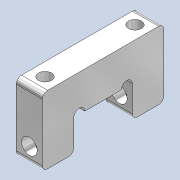
# Autodesk Inventor part: ウィング土台
Saved by Autodesk Inventor 2020 (Build 240168000, 168)
## iProperties
Created: 2020-10-30
Part Number: ウィング土台
Material: アルミニウム 2014-T4
Document SubType Name: Modeling
Designer: AA19065
Density: 2.8 g/cm^3
Appearance: サテン
Author: AA19065
Autodesk Inventor part; units mm, degrees
ref_plane "YZ Plane" through (0, 0, 0) normal (1, 0, 0) x (0, 1, 0)
ref_plane "XZ Plane" through (0, 0, 0) normal (0, 1, 0) x (-1, 0, 0)
ref_plane "XY Plane" through (0, 0, 0) normal (0, 0, 1) x (1, 0, 0)
sketch "スケッチ1" plane through (0, 0, 0) normal (1, 0, 0) x (0, 1, 0)
  line L0 (7, 5.6) -> (0, 5.6)
  line L1 (0, 5.6) -> (0, -5.6)
  line L2 (0, -5.6) -> (7, -5.6)
  line L3 (7, -5.6) -> (7, 5.6)
  line L4 (7, 5.6) -> (-6, 5.6)
  line L5 (-6, 5.6) -> (-6, 13.6)
  line L6 (-6, 13.6) -> (7, 13.6)
  line L7 (7, 13.6) -> (7, 5.6)
  line L8 (7, -5.6) -> (-6, -5.6)
  line L9 (-6, -5.6) -> (-6, -13.6)
  line L10 (-6, -13.6) -> (7, -13.6)
  line L11 (7, -13.6) -> (7, -5.6)
  arc A0 (0, 3.5) -> (0, 5.6) centre (0, 4.55) ccw
  arc A1 (0, -5.6) -> (0, -3.5) centre (0, -4.55) ccw
  point P0 (0, 0)
  point P1 (0, 0)
  point P2 (0, 5.6)
  point P3 (0, 5.6)
  dimension "d0" = 7
  dimension "d1" = 11.2
  dimension "d2" = 13
  dimension "d3" = 13
  dimension "d4" = 8
  dimension "d5" = 8
  dimension "d8" = 1.05
  constraints: 24 end point, 6 parallel, 4 point on circle, 3 horizontal, 3 perpendicular, 2 centre point, 2 point on line, 2 tangent, 1 coincident, 1 equal radius, 1 midpoint
  measures "d0" distance of L2.end L1.end
  measures "d1" distance of L1.end L0.end
  measures "d2" distance of L5.end L6.end
  measures "d3" distance of L10.end L9.end
  measures "d4" distance of L4.end L5.end
  measures "d5" distance of L8.end L9.end
  measures "d8" radius of A0
extrude "押し出し1" add sketch "スケッチ1" along normal blind 5 contours L3 L2 A1 L1 A0 L0 | L0 L4 L5 L6 L7 | L11 L10 L9 L8 L2
sketch "スケッチ2" plane through (0, 7, 13.6) normal (0, 1, 0) x (1, 0, 0)
  line L0 (0, 27.2) -> (0, 0) projected
  line L1 (0, 0) -> (5, 0) projected
  line L2 (5, 27.2) -> (5, 0) projected
  line L3 (0, 27.2) -> (5, 27.2) projected
  line L4 (2.5, 0) -> (2.5, 27.2) construction
  circle A0 centre (2.5, 3) radius 1.25
  circle A1 centre (2.5, 24.2) radius 1.25
  point P0 (0, 13.6)
  dimension "d9" = 2.5
  dimension "d10" = 2.5
  dimension "d11" = 3
  dimension "d12" = 3
  constraints: 2 centre point, 2 end point, 2 midpoint, 2 point on line
  measures "d9" diameter of A0
  measures "d10" diameter of A1
  measures "d11" distance from line of L1 A0.centre
  measures "d12" distance from line of L3 A1.centre
extrude "押し出し2" cut sketch "スケッチ2" against normal up to surface (13 mm away) contours A0 | A1
sketch "スケッチ3" plane through (0, -6, 13.6) normal (0, 0, 1) x (1, 0, 0)
  circle A0 centre (2.5, 3) radius 1.5
  line L0 (0, 0) -> (5, 0) projected
  point P0 (0, 6)
  point P1 (2.5, 0)
  dimension "d15" = 3
  dimension "d16" = 3
  constraints: 1 centre point, 1 midpoint, 1 vertical alignment
  measures "d15" diameter of A0
  measures "d16" distance from line of L0 A0.centre
extrude "押し出し3" cut sketch "スケッチ3" against normal up to surface (27.2 mm away)
fillet "フィレット1" radius 1 6 edges at (2.5, 7, 13.6) (2.5, 7, -13.6) (2.5, -6, -5.6) (2.5, -6, -13.6) (2.5, -6, 5.6) (2.5, -6, 13.6)
equation "\"d3\" = d2"
equation "\"d5\" = d4"
equation "\"d10\" = d9"
equation "\"d12\" = d11"
